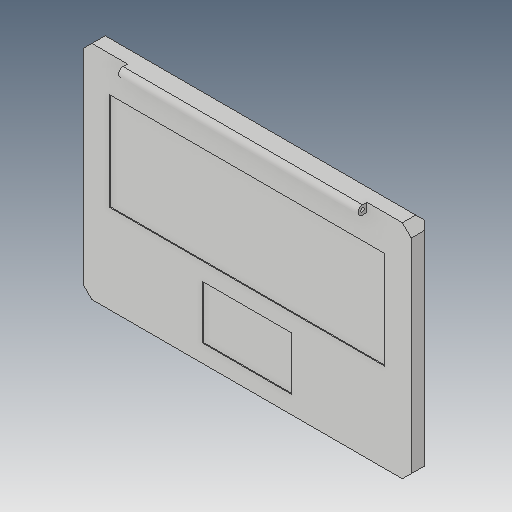
# Autodesk Inventor part: PCパーツ1
Saved by Autodesk Inventor 2020.3 (Build 243373000, 373)
## iProperties
Part Number: PCパーツ1
Material: 一般
Document SubType Name: Modeling
Designer: highs
Density: 1 g/cm^3
Appearance: 既定
Author: highs
Autodesk Inventor part; units mm, degrees
ref_plane "YZ Plane" through (0, 0, 0) normal (1, 0, 0) x (0, 1, 0)
ref_plane "XZ Plane" through (0, 0, 0) normal (0, 1, 0) x (-1, 0, 0)
ref_plane "XY Plane" through (0, 0, 0) normal (0, 0, 1) x (1, 0, 0)
sketch "スケッチ1" plane through (0, 0, 0) normal (0, 0, 1) x (1, 0, 0)
  line L0 (0, 0) -> (370, 0)
  line L1 (370, 0) -> (370, 250)
  line L2 (370, 250) -> (0, 250)
  line L3 (0, 250) -> (0, 0)
  dimension "d0" = 370
  dimension "d1" = 250
  constraints: 8 end point, 2 parallel, 1 horizontal, 1 perpendicular
  measures "d0" distance of L0.start L0.end
  measures "d1" distance of L2.end L0.start
extrude "押し出し1" add sketch "スケッチ1" along normal blind 30
sketch "スケッチ2" plane through (0, 0, 30) normal (0, 0, 1) x (1, 0, 0)
  line L0 (370, 250) -> (0, 250) projected
  line L1 (50, 250) -> (320, 250)
  line L2 (320, 250) -> (320, 240)
  line L3 (320, 240) -> (50, 240)
  line L4 (50, 240) -> (50, 250)
  line L5 (0, 250) -> (0, 0) projected
  line L6 (370, 0) -> (370, 250) projected
  dimension "d4" = 50
  dimension "d5" = 50
  dimension "d6" = 10
  constraints: 8 end point, 2 parallel, 1 horizontal, 1 perpendicular, 1 point on line
  measures "d4" distance between parallel lines of L5 L4
  measures "d5" distance between parallel lines of L6 L2
  measures "d6" distance of L1.end L2.end
extrude "押し出し2" add sketch "スケッチ2" along normal blind 10
fillet "フィレット1" radius 5 2 edges at (185, 240, 40) (185, 250, 40)
chamfer "面取り1" distance 15 angle 45 4 edges at (185, 0, 0) (0, 125, 0) (370, 125, 0) (185, 250, 0)
sketch "スケッチ3" plane through (0, 0, 30) normal (0, 0, 1) x (1, 0, 0)
  line L0 (0, 0) -> (370, 0) projected
  line L1 (185, 0) -> (185, 50) construction
  line L2 (135, 20) -> (235, 20)
  line L3 (235, 20) -> (235, 80)
  line L4 (235, 80) -> (135, 80)
  line L5 (135, 80) -> (135, 20)
  line L6 (135, 20) -> (235, 80) construction
  line L7 (235, 20) -> (135, 80) construction
  line L8 (185, 50) -> (185, 155) construction
  line L9 (30, 210) -> (340, 210)
  line L10 (340, 210) -> (340, 100)
  line L11 (340, 100) -> (30, 100)
  line L12 (30, 100) -> (30, 210)
  line L13 (30, 210) -> (340, 100) construction
  line L14 (340, 210) -> (30, 100) construction
  line L15 (370, 250) -> (320, 250) construction
  line L16 (370, 0) -> (370, 250) construction
  dimension "d13" = 60
  dimension "d14" = 100
  dimension "d15" = 20
  dimension "d16" = 20
  dimension "d17" = 40
  dimension "d18" = 30
  constraints: 28 end point, 5 midpoint, 4 parallel, 2 horizontal, 2 perpendicular, 2 vertical
  measures "d13" distance of L2.end L3.end
  measures "d14" distance of L3.end L4.end
  measures "d15" distance between parallel lines of L0 L2
  measures "d16" distance between parallel lines of L4 L11
  measures "d17" distance between parallel lines of L15 L9
  measures "d18" distance between parallel lines of L16 L10
extrude "押し出し3" cut sketch "スケッチ3" against normal blind 1
chamfer "面取り2" distance 10 angle 45 4 edges at (370, 0, 22.5) (0, 0, 22.5) (370, 250, 22.5) (0, 250, 22.5)
sketch "スケッチ4" plane through (320, 240, 30) normal (1, 0, 0) x (0, 0, -1)
  arc A0 (-5, 10) -> (-5, 0) centre (-5, 5) ccw projected
  circle A1 centre (-5, 5) radius 2
  point P0 (30, -240)
  dimension "d24" = 4
  constraints: 1 centre point, 1 coincident
  measures "d24" diameter of A1
extrude "押し出し4" cut sketch "スケッチ4" against normal up to next
